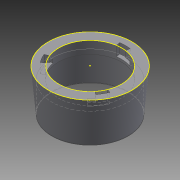
# Autodesk Inventor part: GripScrewCap
Saved by Autodesk Inventor 2014 SP1 (Build 180222100, 222)
## iProperties
Created: 2015-10-17
Part Number: GripScrewCap
Material: Generic
Document SubType Name: Modeling
Designer: anthony
Density: 1 g/cm^3
Appearance: Default
Author: anthony
Autodesk Inventor part; units mm, degrees
ref_plane "YZ Plane" through (0, 0, 0) normal (1, 0, 0) x (0, 1, 0)
ref_plane "XZ Plane" through (0, 0, 0) normal (0, 1, 0) x (-1, 0, 0)
ref_plane "XY Plane" through (0, 0, 0) normal (0, 0, 1) x (1, 0, 0)
sketch "Sketch1" plane through (0, 0, 0) normal (0, 1, 0) x (-1, 0, 0)
  circle A0 centre (0, 0) radius 17
  circle A1 centre (0, 0) radius 12.75
  dimension "d0" = 34
  dimension "d7" = 25.5
  constraints: 2 centre point, 2 coincident
  measures "d0" diameter of A0
  measures "d7" diameter of A1
extrude "Extrusion1" add sketch "Sketch1" along normal blind 5
sketch "Sketch2" plane through (0, 5, 0) normal (0, 1, 0) x (1, 0, 0)
  circle A0 centre (0, 0) radius 12.75 projected
  circle A1 centre (0, 0) radius 17 projected
sketch "Sketch3" plane through (0, 0, 0) normal (0, -1, 0) x (1, 0, 0)
  circle A0 centre (0, 0) radius 17 projected
  circle A1 centre (0, 0) radius 15.5
  dimension "d10" = 31
  constraints: 1 centre point, 1 coincident
  measures "d10" diameter of A1
extrude "Extrusion2" add sketch "Sketch3" along normal blind 12
sketch "Sketch4" plane through (0, 5, 0) normal (0, 1, 0) x (1, 0, 0)
  circle A0 centre (0, 0) radius 12.75 projected
  circle A1 centre (0, 0) radius 17 projected
  line L0 (0, 0) -> (0, 21.0879) construction
  line L1 (0, 0) -> (-3.0708, 20.7306) construction
  line L2 (0, 0) -> (3.1044, 20.9574) construction
  arc A2 (2.1064, 14.2198) -> (-2.1064, 14.2198) centre (0, 0) ccw
  line L3 (-2.1064, 14.2198) -> (-1.8682, 12.6124)
  line L4 (2.1064, 14.2198) -> (1.8682, 12.6124)
  arc A3 (1.8682, 12.6124) -> (-1.8682, 12.6124) centre (0, 0) ccw
  arc A4 (-13.3679, -5.2858) -> (-11.2616, -8.9341) centre (0, 0) ccw
  line L5 (-11.2616, -8.9341) -> (-9.9885, -7.9241)
  line L6 (-13.3679, -5.2858) -> (-11.8568, -4.6882)
  arc A5 (-11.8568, -4.6882) -> (-9.9885, -7.9241) centre (0, 0) ccw
  arc A6 (11.2616, -8.9341) -> (13.3679, -5.2858) centre (0, 0) ccw
  line L7 (13.3679, -5.2858) -> (11.8568, -4.6882)
  line L8 (11.2616, -8.9341) -> (9.9885, -7.9241)
  arc A7 (9.9885, -7.9241) -> (11.8568, -4.6882) centre (0, 0) ccw
  dimension "d14" = 8.426
  dimension "d15" = 8.426
  dimension "d16" = 14.375
  dimension "d21" = 360
  constraints: 18 end point, 14 point on circle, 6 centre point, 4 coincident, 3 point on line, 1 vertical, 31 other
  measures "d14" angle of L1 L0
  measures "d15" angle of L0 L2
  measures "d16" radius of A2
extrude "Extrusion4" cut sketch "Sketch4" against normal blind 4 contours A0 L3 A2 L4 | L7 A6 L8 A0 | A0 L5 A4 L6
sketch "Sketch5" plane through (2.1064, 1, -14.2198) normal (-0.9892063, 0, -0.1465293) x (-0.1465293, 0, 0.9892063)
  line L0 (1.625, 4) -> (1.625, 0) projected
  line L1 (0, 0) -> (1.625, 0)
  line L2 (1.625, 0) -> (1.625, 1.5)
  line L3 (1.625, 1.5) -> (0, 1.5)
  line L4 (0, 1.5) -> (0, 0)
  line L5 (14.375, -16.4) -> (14.375, 7.4) projected
  point P0 (14.375, -1)
  dimension "d26" = 1.5
  constraints: 8 end point, 2 parallel, 1 horizontal, 1 perpendicular, 1 point on line
  measures "d26" distance of L2.end L1.end
revolve "Revolution1" cut sketch "Sketch5" angle 10 about axis through (0, -10, 0) along (0, -1, 0)
sketch "Sketch8" plane through (11.2616, 1, 8.9341) normal (0.6215013, 0, -0.7834131) x (-0.7834131, 0, -0.6215013)
  line L0 (0, 0) -> (2, 0)
  line L1 (2, 0) -> (2, 1.5)
  line L2 (2, 1.5) -> (0, 1.5)
  line L3 (0, 1.5) -> (0, 0)
  line L4 (14.375, -16.4) -> (14.375, 7.4) projected
  point P0 (14, -1)
  point P1 (14.375, 7.4)
  dimension "d28" = 1.5
  constraints: 8 end point, 2 parallel, 1 horizontal, 1 perpendicular, 1 other
  measures "d28" distance of L1.end L0.end
revolve "Revolution2" cut sketch "Sketch8" angle 10 about axis through (0, -10, 0) along (0, -1, 0)
sketch "Sketch9" plane through (-13.3679, 1, 5.2858) normal (0.367705, 0, 0.9299425) x (0.9299425, 0, -0.367705)
  line L0 (0, 0) -> (2, 0)
  line L1 (2, 0) -> (2, 1.5)
  line L2 (2, 1.5) -> (0, 1.5)
  line L3 (0, 1.5) -> (0, 0)
  line L4 (14.375, -16.4) -> (14.375, 7.4) projected
  point P0 (14, -1)
  point P1 (14.375, 7.4)
  dimension "d30" = 1.5
  constraints: 8 end point, 2 parallel, 1 horizontal, 1 perpendicular, 1 other
  measures "d30" distance of L1.end L0.end
revolve "Revolution3" cut sketch "Sketch9" angle 10 about axis through (0, -10, 0) along (0, -1, 0)
draft "FaceDraft1" angle -5 pull direction (0, 1, 0) faces at (-16.9449, 3.3333, -1.3679) (16.9449, -8, -1.3679) fixed edges at (17, 5, 0)
fillet "Fillet1" radius 2 1 edges at (15.5127, -12, 0)
equation "\"d0\" = d3"
equation "\"d14\" = cap_slot_rebate_angle"
equation "\"d15\" = cap_slot_rebate_angle"
equation "\"d16\" = cap_slot_rebate_depth_radius"
equation "\"d23\" = cap_slot_rebate_depth"
equation "\"l1\" = 132"
equation "\"d1\" = 23.5"
equation "\"d3\" = 34"
equation "\"d4\" = 23.5"
equation "\"d5\" = 19"
equation "\"d6\" = 2.2"
equation "\"rco0\" = 13.375"
equation "\"rcod0\" = 12deg"
equation "\"rebate_arc\" = 5"
equation "\"rebate_arc_angle\" = 4.774648deg"
equation "\"rebate_depth\" = 8"
equation "\"min_wall_thickness\" = 1"
equation "\"cap_slot_rebate_angle\" = 8.42585deg"
equation "\"cap_slot_rebate_depth_radius\" = 14.375"
equation "\"cap_slot_rebate_depth\" = 4"
body "Solid1"
